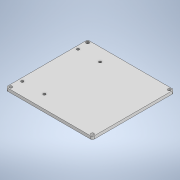
# Autodesk Inventor part: 00_BottomPart
Saved by Autodesk Inventor 2021.1 (Build 251245010, 245A)
## iProperties
Created: 2025-08-17
Part Number: 00_BottomPart
Material: Generic
Document SubType Name: Modeling
Designer: TUAN PC
Density: 1 g/cm^3
Appearance: Default
Author: TUAN PC
Autodesk Inventor part; units mm, degrees
ref_plane "YZ Plane" through (0, 0, 0) normal (1, 0, 0) x (0, 1, 0)
ref_plane "XZ Plane" through (0, 0, 0) normal (0, 1, 0) x (-1, 0, 0)
ref_plane "XY Plane" through (0, 0, 0) normal (0, 0, 1) x (1, 0, 0)
sketch "Base" plane through (0, 0, 0) normal (0, 1, 0) x (-1, 0, 0)
  line L0 (0, 0) -> (-117, 0)
  line L1 (-117, 0) -> (-117, -85)
  line L2 (-117, -85) -> (0, -85)
  line L3 (0, -85) -> (0, 0)
  line L4 (-117, -85) -> (-112, -85)
  line L5 (-112, -85) -> (-112, 0)
  line L6 (-112, 0) -> (-117, 0)
  line L7 (-117, 0) -> (-117, -85)
  circle A0 centre (-114.5, -82.5) radius 1.55
  circle A1 centre (-114.5, -2.5) radius 1.55
  line L8 (-112, -85) -> (-57, -85)
  line L9 (-57, -85) -> (-57, 0)
  line L10 (-57, 0) -> (-112, 0)
  line L11 (-112, 0) -> (-112, -85)
  line L12 (-57, -75) -> (-27, -75)
  line L13 (-27, -75) -> (-27, -10)
  line L14 (-27, -10) -> (-57, -10)
  line L15 (-57, -10) -> (-57, -75)
  circle A2 centre (-30.5, -71.5) radius 1.3
  circle A3 centre (-53.5, -71.5) radius 1.3
  circle A4 centre (-30.5, -13.5) radius 1.3
  circle A5 centre (-53.5, -13.5) radius 1.3
  line L16 (-27, -85) -> (-27, 0)
  circle A6 centre (-29.5, -2.5) radius 1.55
  circle A7 centre (-29.5, -82.5) radius 1.55
  point P0 (-27, -10)
  dimension "d0" = 117
  dimension "d1" = 85
  dimension "d2" = 5
  dimension "d3" = 85
  dimension "d4" = 3.1
  dimension "d5" = 3.1
  dimension "d6" = 2.5
  dimension "d7" = 2.5
  dimension "d8" = 2.5
  dimension "d9" = 2.5
  dimension "d10" = 55
  dimension "d11" = 85
  dimension "d12" = 30
  dimension "d13" = 65
  dimension "d14" = 10
  dimension "d15" = 10
  dimension "d16" = 2.6
  dimension "d17" = 2.6
  dimension "d18" = 2.6
  dimension "d19" = 2.6
  dimension "d20" = 3.5
  dimension "d21" = 3.5
  dimension "d22" = 3.5
  dimension "d23" = 3.5
  dimension "d24" = 3.5
  dimension "d25" = 3.5
  dimension "d26" = 3.5
  dimension "d27" = 3.5
  dimension "d28" = 0
  dimension "d29" = 3.1
  dimension "d30" = 2.5
  dimension "d31" = 2.5
  dimension "d32" = 3.1
  dimension "d33" = 2.5
  dimension "d34" = 2.5
  constraints: 34 end point, 8 centre point, 8 parallel, 5 perpendicular, 4 horizontal, 3 point on line
  measures "d0" distance of L2.end L1.end
  measures "d1" distance of L1.end L0.end
  measures "d2" distance of L6.end L5.end
  measures "d3" distance of L5.end L4.end
  measures "d4" diameter of A0
  measures "d5" diameter of A1
  measures "d6" distance from line of L1 A1.centre
  measures "d7" distance from line of L0 A1.centre
  measures "d8" distance from line of L2 A0.centre
  measures "d9" distance from line of L1 A0.centre
  measures "d10" distance of L10.end L9.end
  measures "d11" distance of L9.end L8.end
  measures "d12" distance of L14.end L13.end
  measures "d13" distance of L13.end L12.end
  measures "d14" distance between parallel lines of L2 L12
  measures "d15" distance between parallel lines of L0 L14
  measures "d16" diameter of A2
  measures "d17" diameter of A3
  measures "d18" diameter of A4
  measures "d19" diameter of A5
  measures "d20" distance from line of L14 A4.centre
  measures "d21" distance from line of L14 A5.centre
  measures "d22" distance from line of L15 A5.centre
  measures "d23" distance from line of L13 A4.centre
  measures "d24" distance from line of L12 A2.centre
  measures "d25" distance from line of L13 A2.centre
  measures "d26" distance from line of A3.centre L15
  measures "d27" distance from line of L12 A3.centre
  measures "d28" distance between parallel lines of L16 L13
  measures "d29" diameter of A6
  measures "d30" distance from line of L16 A6.centre
  measures "d31" distance from line of L0 A6.centre
  measures "d32" diameter of A7
  measures "d33" distance from line of L2 A7.centre
  measures "d34" distance from line of L16 A7.centre
extrude "Extrusion1" add sketch "Base" along normal blind 3 contours L16 L14 L9 L0 | L9 L2 L5 L0 | L13 L12 L9 L14 | L2 L9 L12 L16 | L5 L2 L1 L0
fillet "Fillet1" radius 2 4 edges at (27, 1.5, -85) (117, 1.5, -85) (117, 1.5, 0) (27, 1.5, 0)
body "Solid1"
